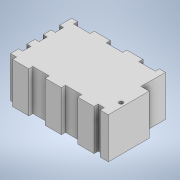
# Autodesk Inventor part: Burrow_Side_Detachable_EXT
Saved by Autodesk Inventor 2020.4 (Build 244396010, 396A)
## iProperties
Created: 2021-09-27
Part Number: Burrow_Side_Detachable_EXT
Material: Generic
Document SubType Name: Sheet Metal
Designer: YUSTE
Density: 1 g/cm^3
Sheet Metal Rule: Default
Appearance: Default
Author: YUSTE
Autodesk Inventor part; units mm, degrees
ref_plane "YZ Plane" through (0, 0, 0) normal (1, 0, 0) x (0, 1, 0)
ref_plane "XZ Plane" through (0, 0, 0) normal (0, 1, 0) x (-1, 0, 0)
ref_plane "XY Plane" through (0, 0, 0) normal (0, 0, 1) x (1, 0, 0)
sketch "Sketch1" plane through (0, 0, 0) normal (0, 1, 0) x (-1, 0, 0)
  line L0 (147.3507, -5.6443) -> (74.3257, -5.6443)
  line L1 (74.3257, -5.6443) -> (74.3257, 45.1557)
  line L2 (74.3257, 45.1557) -> (147.3507, 45.1557)
  line L3 (147.3507, 45.1557) -> (147.3507, -5.6443)
  line L4 (147.3507, 45.1557) -> (142.5882, 45.1557)
  line L5 (142.5882, 45.1557) -> (142.5882, 41.9807)
  line L6 (142.5882, 41.9807) -> (147.3507, 41.9807)
  line L7 (147.3507, 41.9807) -> (147.3507, 45.1557)
  line L8 (129.8882, 45.1557) -> (117.1882, 45.1557)
  line L9 (117.1882, 45.1557) -> (117.1882, 41.9807)
  line L10 (117.1882, 41.9807) -> (129.8882, 41.9807)
  line L11 (129.8882, 41.9807) -> (129.8882, 45.1557)
  line L12 (104.4882, 45.1557) -> (91.7882, 45.1557)
  line L13 (91.7882, 45.1557) -> (91.7882, 41.9807)
  line L14 (91.7882, 41.9807) -> (104.4882, 41.9807)
  line L15 (104.4882, 41.9807) -> (104.4882, 45.1557)
  line L16 (147.3507, -2.4693) -> (147.3507, -5.6443)
  line L17 (129.8882, -5.6443) -> (117.1882, -5.6443)
  line L18 (104.4882, -5.6443) -> (91.7882, -5.6443)
  line L19 (147.3507, 3.8807) -> (147.3507, 10.2307)
  line L20 (147.3507, 10.2307) -> (144.1757, 10.2307)
  line L21 (144.1757, 10.2307) -> (144.1757, 3.8807)
  line L22 (144.1757, 3.8807) -> (147.3507, 3.8807)
  line L23 (147.3507, 16.5807) -> (147.3507, 22.9307)
  line L24 (147.3507, 22.9307) -> (144.1757, 22.9307)
  line L25 (144.1757, 22.9307) -> (144.1757, 16.5807)
  line L26 (144.1757, 16.5807) -> (147.3507, 16.5807)
  line L27 (147.3507, 29.2807) -> (147.3507, 35.6307)
  line L28 (147.3507, 35.6307) -> (144.1757, 35.6307)
  line L29 (144.1757, 35.6307) -> (144.1757, 29.2807)
  line L30 (144.1757, 29.2807) -> (147.3507, 29.2807)
  circle A0 centre (71.1507, 32.0747) radius 1.524
  line L31 (74.3257, 45.1557) -> (79.0882, 45.1557)
  line L32 (79.0882, 45.1557) -> (79.0882, 41.9807)
  line L33 (79.0882, 41.9807) -> (74.3257, 41.9807)
  line L34 (74.3257, 41.9807) -> (74.3257, 45.1557)
  line L35 (74.3257, -2.4693) -> (74.3257, -5.6443)
  line L36 (79.0882, -5.6443) -> (79.0882, -2.4693)
  line L37 (79.0882, -2.4693) -> (91.7882, -2.4693)
  line L38 (91.7882, -2.4693) -> (91.7882, -5.6443)
  line L39 (91.7882, -5.6443) -> (79.0882, -5.6443)
  line L40 (104.4882, -2.4693) -> (104.4882, -5.6443)
  line L41 (104.4882, -5.6443) -> (117.1882, -5.6443)
  line L42 (117.1882, -5.6443) -> (117.1882, -2.4693)
  line L43 (117.1882, -2.4693) -> (104.4882, -2.4693)
  line L44 (129.8882, -5.6443) -> (129.8882, -2.4693)
  line L45 (129.8882, -2.4693) -> (142.5882, -2.4693)
  line L46 (142.5882, -2.4693) -> (142.5882, -5.6443)
  line L47 (142.5882, -5.6443) -> (129.8882, -5.6443)
  line L48 (74.3257, 45.1557) -> (74.3257, 13.4057)
  line L49 (74.3257, 13.4057) -> (67.9757, 13.4057)
  line L50 (67.9757, 13.4057) -> (67.9757, 45.1557)
  line L51 (67.9757, 45.1557) -> (74.3257, 45.1557)
  point P0 (0, 0)
  point P1 (79.0882, -5.6443)
  point P2 (129.8882, -5.6443)
  point P3 (142.5882, -5.6443)
  point P4 (74.3257, 45.1557)
  dimension "d103" = 73.025
  dimension "d104" = 50.8
  dimension "d105" = 4.7625
  dimension "d106" = 3.175
  dimension "d107" = 12.7
  dimension "d108" = 3.175
  dimension "d109" = 12.7
  dimension "d110" = 3.175
  dimension "d111" = 12.7
  dimension "d112" = 12.7
  dimension "d121" = 6.35
  dimension "d122" = 3.175
  dimension "d123" = 6.35
  dimension "d124" = 3.175
  dimension "d126" = 6.35
  dimension "d127" = 6.35
  dimension "d128" = 3.175
  dimension "d129" = 6.35
  dimension "d131" = 3.048
  dimension "d135" = 4.7625
  dimension "d136" = 3.175
  dimension "d141" = 9.906
  dimension "d146" = 3.175
  dimension "d147" = 12.7
  dimension "d148" = 0
  dimension "d149" = 4.7625
  dimension "d150" = 3.175
  dimension "d151" = 12.7
  dimension "d152" = 12.7
  dimension "d153" = 0
  dimension "d154" = 3.175
  dimension "d155" = 12.7
  dimension "d156" = 12.7
  dimension "d159" = 31.75
  dimension "d160" = 6.35
  dimension "d161" = 0
  dimension "d162" = 0
  dimension "d163" = 3.175
  constraints: 104 end point, 24 parallel, 17 point on line, 14 perpendicular, 2 vertical, 1 centre point, 1 horizontal
  measures "d103" distance of L0.start L0.end
  measures "d104" distance of L0.end L1.end
  measures "d105" distance of L2.end L4.end
  measures "d106" distance of L5.end L4.end
  measures "d107" distance of L8.start L8.end
  measures "d108" distance of L9.end L8.end
  measures "d109" distance of L12.start L12.end
  measures "d110" distance of L13.end L12.end
  measures "d111" distance between parallel lines of L5 L11
  measures "d112" distance between parallel lines of L15 L9
  measures "d121" distance of L19.start L19.end
  measures "d122" distance of L20.end L19.end
  measures "d123" distance of L23.start L23.end
  measures "d124" distance of L24.end L23.end
  measures "d126" distance between parallel lines of L26 L20
  measures "d127" distance of L27.start L27.end
  measures "d128" distance of L28.end L27.end
  measures "d129" distance between parallel lines of L24 L30
  measures "d131" diameter of A0
  measures "d135" distance of L1.end L31.end
  measures "d136" distance of L31.end L32.end
  measures "d141" distance from line of L33 A0.centre
  measures "d146" distance of L36.start L36.end
  measures "d147" distance of L36.end L37.end
  measures "d148" distance between parallel lines of L0 L39
  measures "d149" distance between parallel lines of L1 L36
  measures "d150" distance of L40.start L40.end
  measures "d151" distance of L41.end L40.end
  measures "d152" distance between parallel lines of L38 L40
  measures "d153" distance between parallel lines of L0 L41
  measures "d154" distance of L44.start L44.end
  measures "d155" distance of L44.end L45.end
  measures "d156" distance between parallel lines of L42 L44
  measures "d159" distance of L48.start L48.end
  measures "d160" distance of L48.end L49.end
  measures "d161" distance between parallel lines of L1 L48
  measures "d162" distance between parallel lines of L2 L51
  measures "d163" distance from line of L50 A0.centre
extrude "Extrusion10" add sketch "Sketch1" along normal blind 31.75 contours L0 L46 L45 L44 L42 L43 L40 L38 L37 L36 L1 L33 L32 L2 L13 L14 L15 L9 L10 L11 L5 L6 L3 L28 L29 L30 L24 L25 L26 L20 L21 L22 | L49 L50 L51 L1
equation "\"BendRadius\" = Thickness"
equation "\"BendReliefWidth\" = Thickness"
equation "\"BendReliefDepth\" = 0.5 * Thickness"
equation "\"CornerReliefSize\" = 4 * Thickness"
equation "\"MinimumRemnant\" = 2 * Thickness"
equation "\"TransitionRadius\" = BendRadius"
equation "\"JacobiRadiusSize\" = BendRadius"
equation "\"GapSize\" = Thickness"
equation "\"Thickness\" = 3.048"
body "Solid12"
